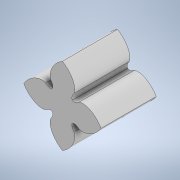
# Autodesk Inventor part: Gear_4t
Saved by Autodesk Inventor 2021 (Build 250183000, 183)
## iProperties
Created: 2021-03-24
Part Number: Gear_4t
Material: Generic
Document SubType Name: Modeling
Designer: lucia
Density: 1 g/cm^3
Appearance: Default
Mass: 110.056 g
Surface Area: 201.589 cm^2
Volume: 110.056 cm^3
Author: lucia
Autodesk Inventor part; units mm, degrees
ref_plane "YZ Plane" through (0, 0, 0) normal (1, 0, 0) x (0, 1, 0)
ref_plane "XZ Plane" through (0, 0, 0) normal (0, 1, 0) x (-1, 0, 0)
ref_plane "XY Plane" through (0, 0, 0) normal (0, 0, 1) x (1, 0, 0)
sketch "Sketch1" plane through (0, 0, 0) normal (0, 0, 1) x (1, 0, 0)
  circle A0 centre (0, 0) radius 26.416
  dimension "d0" = 52.832
  constraints: 1 centre point, 1 coincident
  measures "d0" diameter of A0
extrude "Extrusion1" add sketch "Sketch1" against normal blind 50.8
sketch "Sketch2" plane through (0, 0, 0) normal (0, 0, 1) x (1, 0, 0)
  circle A0 centre (0, 0) radius 13.208
  circle A1 centre (0, 0) radius 26.416
  dimension "d3" = 26.416
  dimension "d4" = 52.832
  constraints: 2 centre point, 2 coincident
  measures "d3" diameter of A0
  measures "d4" diameter of A1
extrude "Extrusion2" cut sketch "Sketch2" against normal blind 50.8
sketch "Sketch3" plane through (0, 0, 0) normal (0, 0, 1) x (1, 0, 0)
  circle A0 centre (0, 0) radius 13.208 projected
  circle A1 centre (0, 0) radius 18.6789
  circle A2 centre (0, 0) radius 13.208
  circle A3 centre (0, 0) radius 26.416
  circle A4 centre (0, 0) radius 39.624
  line L0 (0, 0) -> (10.6636, 15.3359)
  line L1 (0, 0) -> (9.3486, 16.1711)
  line L2 (0, 0) -> (7.9686, 16.8939)
  line L3 (0, 0) -> (6.5331, 17.4992)
  line L4 (0, 0) -> (5.0522, 17.9827)
  line L5 (0, 0) -> (3.5361, 18.3412)
  line L6 (0, 0) -> (1.9954, 18.572)
  line L7 (0, 0) -> (0.4409, 18.6737)
  line L8 (10.6636, 15.3359) -> (9.3486, 16.1711)
  line L9 (9.3486, 16.1711) -> (7.9686, 16.8939)
  line L10 (7.9686, 16.8939) -> (6.5331, 17.4992)
  line L11 (6.5331, 17.4992) -> (5.0522, 17.9827)
  line L12 (5.0522, 17.9827) -> (3.5361, 18.3412)
  line L13 (3.5361, 18.3412) -> (1.9954, 18.572)
  line L14 (1.9954, 18.572) -> (0.4409, 18.6737)
  line L15 (0, 0) -> (-1.1167, 18.6455)
  line L16 (0, 0) -> (-2.6666, 18.4876)
  line L17 (0.4409, 18.6737) -> (-1.1167, 18.6455)
  line L18 (-1.1167, 18.6455) -> (-2.6666, 18.4876)
  line L19 (9.3486, 16.1711) -> (10.6973, 15.3914)
  line L20 (7.9686, 16.8939) -> (10.7865, 15.5647)
  line L21 (5.0522, 17.9827) -> (11.0514, 16.2973)
  line L22 (3.5361, 18.3412) -> (11.1846, 16.8666)
  line L23 (1.9954, 18.572) -> (11.2891, 17.5735)
  line L24 (0.4409, 18.6737) -> (11.3429, 18.4163)
  line L25 (-1.1167, 18.6455) -> (11.3239, 19.3906)
  line L26 (-2.6666, 18.4876) -> (11.2106, 20.4892)
  line L27 (6.5331, 17.4992) -> (10.9115, 15.8646)
  line L28 (0, 0) -> (-4.1979, 18.2011)
  line L29 (0, 0) -> (-5.7, 17.788)
  line L30 (-2.6666, 18.4876) -> (-4.1979, 18.2011)
  line L31 (-4.1979, 18.2011) -> (-5.7, 17.788)
  line L32 (-4.1979, 18.2011) -> (10.9823, 21.7022)
  line L33 (-5.7, 17.788) -> (10.6192, 23.0173)
  line L34 (0, 0) -> (0, 46.5046)
  line L35 (0, 0) -> (9.3395, 9.3395)
  line L36 (0, 0) -> (-7.1624, 17.2512)
  line L37 (-8.575, 16.5943) -> (0, 0)
  line L38 (0, 0) -> (-9.928, 15.822)
  line L39 (0, 0) -> (-11.2119, 14.9397)
  line L40 (0, 0) -> (-12.4179, 13.9535)
  line L41 (0, 0) -> (-13.5374, 12.8702)
  line L42 (-5.7, 17.788) -> (-7.1624, 17.2512)
  line L43 (-7.1624, 17.2512) -> (-8.575, 16.5943)
  line L44 (-8.575, 16.5943) -> (-9.928, 15.822)
  line L45 (-9.928, 15.822) -> (-11.2119, 14.9397)
  line L46 (-11.2119, 14.9397) -> (-12.4179, 13.9535)
  line L47 (-12.4179, 13.9535) -> (-13.5374, 12.8702)
  line L48 (-7.1624, 17.2512) -> (10.103, 24.4195)
  line L49 (-8.575, 16.5943) -> (9.417, 25.8916)
  line L50 (-9.928, 15.822) -> (8.5463, 27.4143)
  line L51 (-11.2119, 14.9397) -> (7.4782, 28.9662)
  line L52 (-12.4179, 13.9535) -> (6.2022, 30.5243)
  line L53 (-13.5374, 12.8702) -> (4.7104, 32.064)
  line L54 (0, 0) -> (-14.5628, 11.6973)
  line L55 (-15.4869, 10.4431) -> (0, 0)
  line L56 (0, 0) -> (-16.3032, 9.1163)
  line L57 (-13.5374, 12.8702) -> (-14.5628, 11.6973)
  line L58 (-14.5628, 11.6973) -> (-15.4869, 10.4431)
  line L59 (-15.4869, 10.4431) -> (-16.3032, 9.1163)
  line L60 (-14.5628, 11.6973) -> (2.9977, 33.5596)
  line L61 (-15.4869, 10.4431) -> (1.0618, 34.9843)
  line L62 (-16.3032, 9.1163) -> (-1.0968, 36.3109)
  spline S0 degree 4 poles (10.6636, 15.3359) (10.6862, 15.3687) (10.7829, 15.5378) (10.9124, 15.8386) (11.0795, 16.3649) (11.208, 16.9327) (11.3098, 17.6413) (11.3599, 18.4847) (11.3376, 19.4603) (11.2207, 20.5598) (10.9887, 21.7738) (10.6218, 23.0898) (10.1017, 24.4928) (9.4117, 25.9655) (8.5368, 27.4887) (7.4643, 29.0409) (6.1839, 30.5991) (4.0875, 32.756) (2.0443, 34.3898) (0.2665, 35.5488) (-1.0968, 36.3109) knots 0 0 0 0 0 0.048321 0.076796 0.109964 0.147188 0.188047 0.232233 0.279505 0.329671 0.382571 0.438068 0.496045 0.556398 0.619039 0.683884 0.750862 0.819906 1 1 1 1 1
  line L63 (10.109, 24.4052) -> (0, 0)
  line L64 (9.3395, 9.3395) -> (7.6611, 11.0178) construction
  line L65 (7.6611, 11.0178) -> (10.6636, 15.3359) construction
  spline S1 degree 2 poles (9.3395, 9.3395) (7.6611, 11.0178) (10.6636, 15.3359) knots 1 1 1 2 2 2
  line L66 (0, 0) -> (-10.6636, 15.3359)
  spline S2 degree 4 poles (-10.6636, 15.3359) (-10.6862, 15.3687) (-10.7829, 15.5378) (-10.9124, 15.8386) (-11.0795, 16.3649) (-11.208, 16.9327) (-11.3098, 17.6413) (-11.3599, 18.4847) (-11.3376, 19.4603) (-11.2207, 20.5598) (-10.9887, 21.7738) (-10.6218, 23.0898) (-10.1017, 24.4928) (-9.4117, 25.9655) (-8.5368, 27.4887) (-7.4643, 29.0409) (-6.1839, 30.5991) (-4.0875, 32.756) (-2.0443, 34.3898) (-0.2665, 35.5488) (1.0968, 36.3109) knots 0 0 0 0 0 0.048321 0.076796 0.109964 0.147188 0.188047 0.232233 0.279505 0.329671 0.382571 0.438068 0.496045 0.556398 0.619039 0.683884 0.750862 0.819906 1 1 1 1 1
  line L67 (-9.3395, 9.3395) -> (-7.6611, 11.0178) construction
  line L68 (-7.6611, 11.0178) -> (-10.6636, 15.3359) construction
  spline S3 degree 2 poles (-9.3395, 9.3395) (-7.6611, 11.0178) (-10.6636, 15.3359) knots 1 1 1 2 2 2
  point P0 (7.5403, 10.8441)
  point P1 (-7.928, 10.564)
  point P2 (-10.6973, 15.3914)
  point P3 (-10.7865, 15.5647)
  point P4 (-11.0514, 16.2973)
  point P5 (-11.1846, 16.8666)
  point P6 (-11.2891, 17.5735)
  point P7 (-11.3429, 18.4163)
  point P8 (-11.3239, 19.3906)
  point P9 (-11.2106, 20.4892)
  point P10 (-10.9115, 15.8646)
  point P11 (-10.9823, 21.7022)
  point P12 (-10.6192, 23.0173)
  point P13 (-10.103, 24.4195)
  point P14 (-9.417, 25.8916)
  point P15 (-8.5463, 27.4143)
  point P16 (-7.4782, 28.9662)
  point P17 (-6.2022, 30.5243)
  point P18 (-4.7104, 32.064)
  point P19 (-2.9977, 33.5596)
  point P20 (-1.0618, 34.9843)
  point P21 (0, 35.6678)
  dimension "d8" = 52.832
  dimension "d9" = 26.416
  dimension "d10" = 37.3579
  dimension "d7" = 79.248
  dimension "d11" = 1.5579
  dimension "d12" = 1.5579
  dimension "d13" = 3.1157
  dimension "d14" = 4.6736
  dimension "d15" = 6.2315
  dimension "d16" = 7.7893
  dimension "d17" = 9.3472
  dimension "d19" = 10.9051
  dimension "d20" = 12.4629
  dimension "d22" = 14.0208
  dimension "d23" = 15.5787
  dimension "d24" = 17.1365
  dimension "d26" = 45
  dimension "d32" = 18.6944
  dimension "d33" = 20.2523
  dimension "d34" = 21.8101
  dimension "d35" = 23.368
  dimension "d36" = 24.9259
  dimension "d37" = 26.4837
  dimension "d40" = 28.0416
  dimension "d41" = 29.5995
  dimension "d42" = 31.1573
  dimension "d43" = 22.5
  constraints: 102 end point, 23 symmetric about line, 19 equal length, 3 coincident, 2 vertical, 132 other
  measures "d7" diameter of A4
  measures "d11" distance of L8.start L1.end
  measures "d12" distance of L1.end L19.end
  measures "d13" distance of L2.end L20.end
  measures "d14" distance of L3.end L27.end
  measures "d15" distance of L4.end L21.end
  measures "d16" distance of L5.end L22.end
  measures "d17" distance of L6.end L23.end
  measures "d19" distance of L7.end L24.end
  measures "d20" distance of L15.end L25.end
  measures "d22" distance of L16.end L26.end
  measures "d23" distance of L28.end L32.end
  measures "d24" distance of L29.end L33.end
  measures "d26" angle of L34 L35
  measures "d32" distance of L36.end L48.end
  measures "d33" distance of L37.start L49.end
  measures "d34" distance of L38.end L50.end
  measures "d35" distance of L45.end L51.end
  measures "d36" distance of L40.end L52.end
  measures "d37" distance of L41.end L53.end
  measures "d40" distance of L54.end L60.end
  measures "d41" distance of L55.start L61.end
  measures "d42" distance of L56.end L62.end
  measures "d43" angle of L34 L63
extrude "Extrusion3" add sketch "Sketch3" against normal blind 50.8 contours A0 L0 S1 | A0 L1 A1 L0 | A1 L19 S0 | A0 L2 A1 L1 | A0 L63 L10 L2 | L3 L10 L63 A0 | A0 L4 L11 L3 | A0 L5 L12 L4 | A0 L6 A1 L5 | A0 L7 A1 L6 | A0 L34 L17 L7 | L15 L17 L34 A0 | A0 L16 L18 L15 | A0 L28 L30 L16 | A0 L29 L31 L28 | A0 L36 L42 L29 | A0 L37 L43 L36 | A0 L38 A1 L37 | A0 L66 L45 L38 | L39 S3 L66 A0 | A0 L40 S3 L39 | A0 S3 L40 | A1 L20 S0 L19 | S2 A3 L62 | L62 A3 L61 S2 | L10 L63 A1 | A1 L63 L27 S0 L20 | L11 A1 | L27 L63 A1 | A1 L63 L10 | A1 L21 L63 L27 | L12 A1 | A1 L22 L63 L21 | A1 L23 L63 L22 | A1 L24 L63 L23 | L17 L34 A1 | A1 L34 L25 L63 L24 | L18 A1 | L25 L34 A1 | A1 L34 L17 | A1 L26 L34 L25 | L30 A1 | A1 L32 L34 L26 | L31 A1 | A1 L33 L34 L32 | L42 A1 | A1 L48 L34 L33 | L43 A1 | A1 L49 L34 L48 | A1 L50 L34 L49 | L45 L66 A1 | A1 S2 L51 L34 L50 | L61 A3 L60 S2 | L62 S2 L34 L61 A3 | A3 S2 L62 | L63 L21 S0 L27 | L63 L22 S0 L21 | L63 L23 S0 L22 | L63 L24 S0 L23 | L63 L25 S0 L24 | L34 L26 L63 L25 | L34 L32 L63 L26 | L34 L33 L63 L32 | L34 L48 A3 L63 L33 | L34 L49 A3 L48 | L34 L50 A3 L49 | L34 L51 A3 L50 | S2 L60 A3 L53 | L53 A3 L34 L52 S2 | L61 L34 L60 A3 | L63 L26 S0 L25 | L63 L32 S0 L26 | L63 L33 S0 L32 | L63 S0 L33 | L48 S0 A3 | A3 L49 S0 L48 | A3 L50 S0 L49 | S2 L52 L34 L51 | L34 L52 A3 L51 | A3 L51 S0 L50 | L53 L34 A3 | A3 L60 L34 L53 | L61 S0 L60 L34 | L34 S0 L61 | L34 A3 L52 | A3 L52 S0 L51 | L34 L53 S0 L52 A3 | L34 L60 S0 L53 picked at (-10.2527, 15.6029)
pattern_circular "Circular Pattern1" count 4 over 360 about axis through (0, 0, 0) along (0, 0, -1) of "Extrusion3"
equation "\"d0\" = 13.208 * scale"
equation "\"d1\" = 12.7 * scale"
equation "\"d3\" = 6.604 * scale"
equation "\"d4\" = 13.208 * scale"
equation "\"d5\" = 12.7 * scale"
equation "\"d8\" = 13.208 * scale"
equation "\"d9\" = 6.604 * scale"
equation "\"d10\" = 9.33947 * scale"
equation "\"d7\" = 19.812 * scale"
equation "\"d27\" = 12.7 * scale"
equation "\"prcsn\" = 0.38947"
equation "\"scale\" = 4"
body "Solid1"
